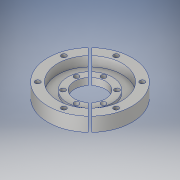
# Autodesk Inventor part: heatsink
Saved by Autodesk Inventor 2018 (Build 220112000, 112)
## iProperties
Created: 2019-03-04
Part Number: heatsink
Material: Aluminum 6061
Document SubType Name: Modeling
Designer: Admin
Density: 2.7 g/cm^3
Appearance: Aluminum - Flat
Author: Admin
Autodesk Inventor part; units mm, degrees
ref_plane "YZ Plane" through (0, 0, 0) normal (1, 0, 0) x (0, 1, 0)
ref_plane "XZ Plane" through (0, 0, 0) normal (0, 1, 0) x (-1, 0, 0)
ref_plane "XY Plane" through (0, 0, 0) normal (0, 0, 1) x (1, 0, 0)
sketch "Sketch1" plane through (0, 0, 0) normal (0, 1, 0) x (-1, 0, 0)
  circle A0 centre (0, 0) radius 13.97
  circle A1 centre (0, 0) radius 38.1
  dimension "d0" = 27.94
  dimension "d1" = 76.2
  constraints: 2 centre point, 2 coincident
  measures "d0" diameter of A0
  measures "d1" diameter of A1
extrude "Extrusion1" add sketch "Sketch1" along normal blind 12.7
sketch "Sketch2" plane through (0, 12.7, 0) normal (0, 1, 0) x (1, 0, 0)
  circle A0 centre (0, 0) radius 20.32
  circle A1 centre (0, 0) radius 13.97 projected
  circle A2 centre (0, 0) radius 29.21
  circle A3 centre (0, 0) radius 38.1 projected
  dimension "d4" = 6.35
  dimension "d63" = 58.42
  constraints: 2 centre point, 2 coincident
  measures "d4" radial gap between concentric circles of A0 A1
  measures "d63" diameter of A2
extrude "Extrusion2" cut sketch "Sketch2" against normal blind 8.89 contours A2
sketch "Sketch3" plane through (0, 12.7, 0) normal (0, 1, 0) x (1, 0, 0)
  line L0 (0, 0) -> (12.2131, 12.2131) construction
  line L1 (0, 0) -> (17.272, 0) construction
  dimension "d7" = 17.272
  dimension "d8" = 45
  constraints: 4 end point, 1 coincident, 1 equal length, 1 horizontal
  measures "d7" distance of L0.start L0.end
  measures "d8" angle of L1 L0
hole "Hole1" at (12.2131, 12.7, -12.2131) direction (0, -1, 0) diameter 4.4958 depth 25.4 tip angle 118 clearance for "Flat Head Machine Screw (82)" size "#8" standard "Ansi Unified Screw Threads"
pattern_circular "Circular Pattern1" count 6 over 360 about axis through (0, 0, 0) along (0, 1, 0) of "Hole1"
sketch "Sketch8" plane through (0, 12.7, 0) normal (0, 1, 0) x (1, 0, 0)
  circle A0 centre (0, 0) radius 20.32
  circle A1 centre (0, 0) radius 20.32 projected
  constraints: 1 centre point, 1 coincident, 1 concentric
extrude "Extrusion5" cut sketch "Sketch8" against normal blind 6.35
sketch "Sketch9" plane through (0, 12.7, 0) normal (0, 1, 0) x (1, 0, 0)
  circle A0 centre (0, 0) radius 38.1 construction
  circle A1 centre (0, 0) radius 38.1 construction
  circle A2 centre (0, 0) radius 33.528 construction
  line L0 (0, 0) -> (23.7079, 23.7079) construction
  line L1 (0, 0) -> (33.528, 0) construction
  dimension "d47" = 4.572
  dimension "d48" = 45
  constraints: 4 end point, 3 coincident, 1 centre point, 1 concentric, 1 equal length, 1 horizontal, 3 other
  measures "d48" angle of L1 L0
hole "Hole3" at (23.7079, 12.7, -23.7079) direction (0, -1, 0) diameter 4.4958 depth 25.4 tip angle 118 clearance for "Flat Head Machine Screw (82)" size "#8" standard "Ansi Unified Screw Threads"
pattern_circular "Circular Pattern3" count 6 over 360 about axis through (0, 0, 0) along (0, 1, 0) of "Hole3"
sketch "Sketch10" plane through (0, 12.7, 0) normal (0, 1, 0) x (1, 0, 0)
  line L0 (27.8388, -26.0427) -> (-26.0427, 27.8388)
  line L1 (-26.0427, 27.8388) -> (-27.8388, 26.0427)
  line L2 (-27.8388, 26.0427) -> (26.0427, -27.8388)
  line L3 (26.0427, -27.8388) -> (27.8388, -26.0427)
  line L4 (27.8388, -26.0427) -> (-27.8388, 26.0427) construction
  line L5 (-26.0427, 27.8388) -> (26.0427, -27.8388) construction
  line L6 (27.8388, -26.0427) -> (104.0388, -26.0427) construction
  circle A0 centre (0, 0) radius 38.1 projected
  dimension "d59" = 135
  dimension "d60" = 2.54
  constraints: 14 end point, 2 midpoint, 2 parallel, 1 equal length, 1 horizontal, 1 perpendicular, 1 tangent
  measures "d59" angle of L6 L0
  measures "d60" distance of L1.end L0.end
extrude "Extrusion6" cut sketch "Sketch10" against normal up to surface (12.7 mm away) contours L3 A0 L0 | A0 L2 L0 | L3 L2 A0 | A0 L1 L0 | A0 L2 L1
body "Solid1"
